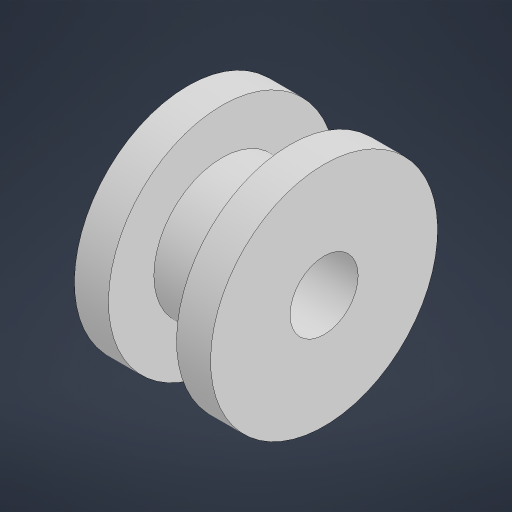
# Autodesk Inventor part: Pulley_D3_P6
Saved by Autodesk Inventor 2024.2 (Build 282272000, 272)
## iProperties
Created: 2024-03-07
Part Number: Pulley_D3_P6
Material: 一般
Document SubType Name: Modeling
Designer: Hanaoka
Density: 1 g/cm^3
Appearance: 既定
Author: Hanaoka
Autodesk Inventor part; units mm, degrees
ref_plane "YZ Plane" through (0, 0, 0) normal (1, 0, 0) x (0, 1, 0)
ref_plane "XZ Plane" through (0, 0, 0) normal (0, 1, 0) x (-1, 0, 0)
ref_plane "XY Plane" through (0, 0, 0) normal (0, 0, 1) x (1, 0, 0)
sketch "スケッチ1" plane through (0, 0, 0) normal (0, 0, 1) x (1, 0, 0)
  line L0 (0, 3) -> (1.5, 3)
  line L1 (1.5, 3) -> (1.5, 5)
  line L2 (1.5, 5) -> (3, 5)
  line L3 (3, 5) -> (3, 1.5)
  line L4 (3, 1.5) -> (-0.0006, 1.5)
  line L5 (0, -1) -> (0, 6) construction
  line L6 (0, 3) -> (-1.5, 3)
  line L7 (-1.5, 3) -> (-1.5, 5)
  line L8 (-1.5, 5) -> (-3, 5)
  line L9 (-3, 5) -> (-3, 1.5)
  line L10 (-3, 1.5) -> (0.0006, 1.5)
  line L11 (-4.2, 0) -> (4.2, 0) projected
  point P0 (0, 0)
  point P1 (-0.0006, 1.5)
  dimension "d0" = 1.5
  dimension "d1" = 3
  dimension "d2" = 1.5
  dimension "d3" = 1.5
  dimension "d4" = 2
  constraints: 20 end point, 5 symmetric about line, 3 perpendicular, 2 horizontal, 1 point on line
  measures "d0" distance of L4.end point (0, 0)
  measures "d1" distance from line of point (0, 0) L0
  measures "d2" distance of L0.start L0.end
  measures "d3" distance of L1.end L2.end
  measures "d4" distance of L0.end L1.end
revolve "回転1" add sketch "スケッチ1" angle 360 about axis through (-10, 0, 0) along (1, 0, 0)
